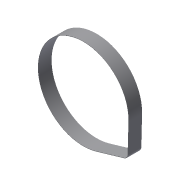
# Autodesk Inventor part: PoleHeightMarker
Saved by Autodesk Inventor 2017 (Build 210142000, 142)
## iProperties
Created: 2017-01-27
Part Number: PoleHeightMarker
Material: Generic
Document SubType Name: Modeling
Designer: krosie
Density: 1 g/cm^3
Appearance: Default
Author: krosie
Autodesk Inventor part; units mm, degrees
ref_plane "YZ Plane" through (0, 0, 0) normal (1, 0, 0) x (0, 1, 0)
ref_plane "XZ Plane" through (0, 0, 0) normal (0, 1, 0) x (-1, 0, 0)
ref_plane "XY Plane" through (0, 0, 0) normal (0, 0, 1) x (1, 0, 0)
sketch "Sketch1" plane through (0, 0, 0) normal (0, 0, 1) x (1, 0, 0)
  circle A0 centre (0, 0) radius 101.6 construction
  arc A1 (78.464, -64.852) -> (82.3203, -59.5483) centre (88.8846, -68.3749) ccw construction
  line L0 (101.5669, -2.5919) -> (99.881, -68.6555)
  line L1 (91.9762, -78.9315) -> (28.5548, -97.5048)
  arc A2 (101.5669, -2.5919) -> (28.5548, -97.5048) centre (0, 0) ccw
  arc A3 (91.9762, -78.9315) -> (99.881, -68.6555) centre (88.8846, -68.3749) ccw
  line L2 (100.6577, -68.6753) -> (102.3436, -2.6117)
  arc A4 (102.3436, -2.6117) -> (28.7731, -98.2504) centre (0, 0) ccw
  line L3 (28.7731, -98.2504) -> (92.1945, -79.6771)
  arc A5 (92.1945, -79.6771) -> (100.6577, -68.6753) centre (88.8846, -68.3749) ccw
  point P0 (0, 0)
  dimension "d0" = 0.7769
  constraints: 12 point on circle, 8 end point, 4 centre point, 4 tangent, 2 coincident, 3 other
  measures "d0" distance between parallel lines of L0 L2
extrude "Extrusion1" add sketch "Sketch1" against normal blind 30
body "Solid1"
